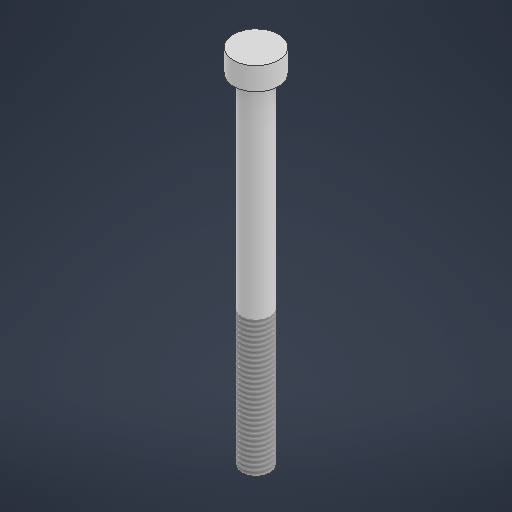
# Autodesk Inventor part: 01-03-05 Schraube
Saved by Autodesk Inventor 2026.2 (Build 302298000, 298)
## iProperties
Created: 2025-12-18
Part Number: 01-03-05 Schraube
Material: Generisch
Document SubType Name: Modeling
Designer: Schally
Density: 1 g/cm^3
Appearance: Vorgabe
Author: Schally
Autodesk Inventor part; units mm, degrees
ref_plane "YZ Plane" through (0, 0, 0) normal (1, 0, 0) x (0, 1, 0)
ref_plane "XZ Plane" through (0, 0, 0) normal (0, 1, 0) x (-1, 0, 0)
ref_plane "XY Plane" through (0, 0, 0) normal (0, 0, 1) x (1, 0, 0)
sketch "Skizze1" plane through (0, 0, 0) normal (1, 0, 0) x (0, 1, 0)
  line L0 (-12.8, 0) -> (76.8, 0) projected
  line L1 (0, -0.8) -> (0, 4.8) projected
  line L2 (0, 0) -> (0, 2.5)
  line L3 (0, 2.5) -> (60, 2.5)
  line L4 (60, 2.5) -> (60, 4)
  line L5 (60, 4) -> (64, 4)
  line L6 (64, 4) -> (64, 0)
  dimension "d0" = 2.5
  dimension "d1" = 60
  dimension "d3" = 4
  dimension "d8" = 4
  constraints: 10 end point, 4 perpendicular, 2 point on line
  measures "d0" distance of L2.start L2.end
  measures "d1" distance of L2.end L3.end
  measures "d3" distance of L4.end L5.end
  measures "d8" distance between parallel lines of L0 L5
revolve "Umdrehung1" add sketch "Skizze1" angle 360 about axis through (0, -10, 0) along (0, 1, 0)
thread "Gewinde1" size "M5x0.8" class "6g" standard "ANSI Metric M Profile" length 24
